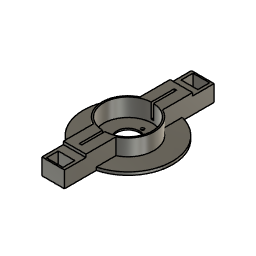
silnik v1 v2 (Autodesk Fusion 360 design; units mm, degrees)
Autodesk Fusion 360 part; units mm, degrees
cylinder "CylinderPrimitive1" add diameter 35 height 1 placed x (1, 0, 0) y (0, 1, 0) z (0, 0, 1) at (0, 0, 0)
cylinder "CylinderPrimitive2" cut diameter 15.2 height -1 placed x (1, 0, 0) y (0, 1, 0) z (0, 0, 1) at (0, 0, 1)
sketch "Sketch3" plane through (0, 0, 1) normal (0, 0, 1) x (-1, 0, 0)
  circle A0 centre (0, 0) radius 7.6
  circle A1 centre (0, 0) radius 17.5
  circle A2 centre (0, 0) radius 17.5
  circle A3 centre (0, 0) radius 16.5
  line L0 (-7.6, -50) -> (7.6, -50)
  line L1 (7.6, -50) -> (7.6, 50)
  line L2 (7.6, 50) -> (-7.6, 50)
  line L3 (-7.6, 50) -> (-7.6, -50)
  dimension "d5" = 33
  dimension "d6" = 15.2
  dimension "d7" = 100
  dimension "d8" = 50
  dimension "d9" = 7.6
  constraint coincident A0.centre A1.centre
  constraint horizontal L0
  constraint vertical L1
  constraint horizontal L2
  constraint vertical L3
  measures "d5" diameter of A3
  measures "d6" distance of L0.start L0.end
  measures "d7" distance of L0.start L2.end
  measures "d8" distance of A0.centre L0
  measures "d9" distance of A0.centre L3
extrude "Extrude1" add sketch "Sketch3" against normal blind 1 contours A1 A2 L1 L2 L3
extrude "Extrude2" add sketch "Sketch3" against normal blind 1 contours A1 A2 L0 L1 L3
extrude "Extrude3" add sketch "Sketch3" along normal blind 10 contours A1 A2 A3 L1 L3 | A1 A2 A3 L1 | A1 A2 A3 L1 L3 | A1 A2 A3 L3
sketch "Sketch4" plane through (0, 0, 1) normal (0, 0, 1) x (-1, 0, 0)
  arc A0 (-7.6, -15.7636) -> (7.6, -15.7636) centre (0, 0) ccw
  line L0 (-7.6, -15.7636) -> (-7.6, -50)
  line L1 (-7.6, -50) -> (7.6, -50)
  line L2 (7.6, -50) -> (7.6, -15.7636)
  line L3 (5.6, -49.5) -> (-5.6, -49.5)
  line L4 (-5.6, -49.5) -> (-5.6, -11)
  line L5 (-5.6, -11) -> (5.6, -11)
  line L6 (5.6, -11) -> (5.6, -49.5)
  line L7 (-7.6, 50) -> (-7.6, 15.7636)
  line L8 (7.6, 15.7636) -> (7.6, 50)
  line L9 (7.6, 50) -> (-7.6, 50)
  dimension "d16" = 2
  dimension "d17" = 2
  dimension "d18" = 0.5
  constraint horizontal L3
  constraint vertical L4
  constraint horizontal L5
  constraint vertical L6
  measures "d16" distance of L2 L6
  measures "d17" distance of L0 L4
  measures "d18" distance of L1 L3
extrude "Extrude4" add sketch "Sketch4" along normal blind 10 contours A0 L0 L1 L2 L3 L4 L6
sketch "Sketch5" plane through (0, 0, 1) normal (0, 0, 1) x (-1, 0, 0)
  arc A0 (7.6, 15.7636) -> (-7.6, 15.7636) centre (0, 0) ccw
  line L0 (7.6, 15.7636) -> (7.6, 50)
  line L1 (7.6, 50) -> (-7.6, 50)
  line L2 (-7.6, 50) -> (-7.6, 15.7636)
  line L3 (-5.6, 49.5) -> (5.6, 49.5)
  line L4 (5.6, 49.5) -> (5.6, 12.5)
  line L5 (5.6, 12.5) -> (-5.6, 12.5)
  line L6 (-5.6, 12.5) -> (-5.6, 49.5)
  dimension "d25" = 2
  dimension "d26" = 2
  dimension "d27" = 0.5
  constraint horizontal L3
  constraint vertical L4
  constraint horizontal L5
  constraint vertical L6
  measures "d25" distance of L2 L6
  measures "d26" distance of L0 L4
  measures "d27" distance of L1 L3
extrude "Extrude5" add sketch "Sketch5" along normal blind 10 contours A0 L0 L1 L2 L3 L4 L6
sketch "Sketch6" plane through (0, 0, 11) normal (0, 0, 1) x (-1, 0, 0)
  arc A0 (5.6, 16.5798) -> (-5.6, 16.5798) centre (0, 0) ccw
  line L0 (-5.6, 16.5798) -> (-5.6, 49.5)
  line L1 (-5.6, 49.5) -> (5.6, 49.5)
  line L2 (5.6, 49.5) -> (5.6, 16.5798)
  arc A1 (-5.6, -16.5798) -> (5.6, -16.5798) centre (0, 0) ccw
  line L3 (5.6, -16.5798) -> (5.6, -49.5)
  line L4 (5.6, -49.5) -> (-5.6, -49.5)
  line L5 (-5.6, -49.5) -> (-5.6, -16.5798)
  circle A2 centre (0, 0) radius 16.5
  line L6 (7.6, 15.7636) -> (7.6, 50)
  line L7 (7.6, 50) -> (-7.6, 50)
  line L8 (-7.6, 50) -> (-7.6, 15.7636)
  arc A3 (-7.6, 15.7636) -> (-7.6, -15.7636) centre (0, 0) ccw
  line L9 (-7.6, -15.7636) -> (-7.6, -50)
  line L10 (-7.6, -50) -> (7.6, -50)
  line L11 (7.6, -50) -> (7.6, -15.7636)
  arc A4 (7.6, -15.7636) -> (7.6, 15.7636) centre (0, 0) ccw
  line L12 (-5.6, 41.5) -> (5.6, 41.5)
  line L13 (5.6, 41.5) -> (5.6, 16.5798)
  line L14 (5.6, 16.5798) -> (-5.6, 16.5798)
  line L15 (-5.6, 16.5798) -> (-5.6, 41.5)
  line L16 (-5.6, -16.5798) -> (5.6, -16.5798)
  line L17 (5.6, -16.5798) -> (5.6, -41.5)
  line L18 (5.6, -41.5) -> (-5.6, -41.5)
  line L19 (-5.6, -41.5) -> (-5.6, -16.5798)
  dimension "d30" = 8
  dimension "d31" = 8
  constraint horizontal L12
  constraint vertical L13
  constraint horizontal L14
  constraint vertical L15
  constraint coincident A0.start L2.end
  constraint coincident L0 L12.start
  constraint horizontal L16
  constraint vertical L17
  constraint horizontal L18
  constraint vertical L19
  constraint coincident L3 L17.end
  constraint coincident A1.start L5.end
  measures "d30" distance of L1 L12
  measures "d31" distance of L4 L18
extrude "Extrude6" add sketch "Sketch6" against normal blind 10 contours A1 L3 L5 L17 L18 L19
extrude "Extrude7" add sketch "Sketch6" against normal blind 10 contours A0 L0 L2 L12 L13 L15
sketch "Sketch7" plane through (0, 0, 11) normal (0, 0, 1) x (-1, 0, 0)
  line L0 (5.6, 41.5) -> (-5.6, 41.5)
  line L1 (-5.6, 41.5) -> (-5.6, 49.5)
  line L2 (-5.6, 49.5) -> (5.6, 49.5)
  line L3 (5.6, 49.5) -> (5.6, 41.5)
  line L4 (5.6, -41.5) -> (5.6, -49.5)
  line L5 (5.6, -49.5) -> (-5.6, -49.5)
  line L6 (-5.6, -49.5) -> (-5.6, -41.5)
  line L7 (-5.6, -41.5) -> (5.6, -41.5)
  circle A0 centre (0, 0) radius 16.5
  line L8 (7.6, 15.7636) -> (7.6, 50)
  line L9 (7.6, 50) -> (-7.6, 50)
  line L10 (-7.6, 50) -> (-7.6, 15.7636)
  arc A1 (-7.6, 15.7636) -> (-7.6, -15.7636) centre (0, 0) ccw
  line L11 (-7.6, -15.7636) -> (-7.6, -50)
  line L12 (-7.6, -50) -> (7.6, -50)
  line L13 (7.6, -50) -> (7.6, -15.7636)
  arc A2 (7.6, -15.7636) -> (7.6, 15.7636) centre (0, 0) ccw
  line L14 (-2.5, -40.5) -> (-0.5, -40.5)
  line L15 (-0.5, -40.5) -> (-0.5, -17)
  line L16 (-0.5, -17) -> (-2.5, -17)
  line L17 (-2.5, -17) -> (-2.5, -40.5)
  line L18 (0.5, -40.5) -> (2.5, -40.5)
  line L19 (2.5, -40.5) -> (2.5, -17)
  line L20 (2.5, -17) -> (0.5, -17)
  line L21 (0.5, -17) -> (0.5, -40.5)
  line L22 (-2.5, 17) -> (-0.5, 17)
  line L23 (-0.5, 17) -> (-0.5, 40.5)
  line L24 (-0.5, 40.5) -> (-2.5, 40.5)
  line L25 (-2.5, 40.5) -> (-2.5, 17)
  line L26 (0.5, 17) -> (2.5, 17)
  line L27 (2.5, 17) -> (2.5, 40.5)
  line L28 (2.5, 40.5) -> (0.5, 40.5)
  line L29 (0.5, 40.5) -> (0.5, 17)
  dimension "d36" = 1
  dimension "d37" = 1
  dimension "d38" = 7.1
  dimension "d39" = 7.1
  dimension "d40" = 1
  dimension "d41" = 17
  dimension "d42" = 17
  dimension "d43" = 17
  dimension "d44" = 1
  dimension "d45" = 1
  constraint horizontal L14
  constraint vertical L15
  constraint horizontal L16
  constraint vertical L17
  constraint horizontal L18
  constraint vertical L19
  constraint horizontal L20
  constraint vertical L21
  constraint horizontal L22
  constraint vertical L23
  constraint horizontal L24
  constraint vertical L25
  constraint horizontal L26
  constraint vertical L27
  constraint horizontal L28
  constraint vertical L29
  measures "d36" distance of L15 L21
  measures "d37" distance of L23 L29
  measures "d38" distance of L11 L15.end
  measures "d39" distance of L10 L23.end
  measures "d40" distance of L0 L24
  measures "d41" distance of A0.centre L22
  measures "d42" distance of A0.centre L26
  measures "d43" distance of A0.centre L16
  measures "d44" distance of L7 L14
  measures "d45" distance of L7 L18
extrude "Extrude8" add sketch "Sketch7" along normal blind 10 contours L14 L15 L16 L17 | L18 L19 L20 L21 | L22 L23 L24 L25 | L26 L27 L28 L29
delete_face "Usuń powierzchnię1" 3 faces at (1.8333, -32.6667, 21) (2.5, -32.6667, 14.3333) (1.1667, -40.5, 14.3333)
delete_face "Usuń powierzchnię2" 2 faces at (-1.8333, -40.5, 17.6667) (-0.5, -32.6667, 14.3333)
delete_face "Usuń powierzchnię3" 3 faces at (2.5, 24.8333, 17.6667) (1.8333, 24.8333, 21) (1.1667, 17, 14.3333)
delete_face "Usuń powierzchnię4" 2 faces at (-0.5, 24.8333, 17.6667) (-1.8333, 17, 17.6667)
sketch "Szkic8" plane through (0, 0, 0) normal (0, 0, 1) x (1, 0, 0)
  circle A0 centre (0, 0) radius 30
  dimension "d48" = 60
  constraint coincident A0.centre origin
  measures "d48" diameter of A0
sketch "Szkic9" plane through (0, 0, 0) normal (0, 0, -1) x (1, 0, 0)
  circle A0 centre (0, 0) radius 7.6
  arc A1 (-7.6, 15.7636) -> (-7.6, -15.7636) centre (0, 0) ccw
  line L0 (-7.6, -15.7636) -> (-7.6, -50)
  line L1 (-7.6, -50) -> (7.6, -50)
  line L2 (7.6, -50) -> (7.6, -15.7636)
  arc A2 (7.6, -15.7636) -> (7.6, 15.7636) centre (0, 0) ccw
  line L3 (7.6, 15.7636) -> (7.6, 50)
  line L4 (7.6, 50) -> (-7.6, 50)
  line L5 (-7.6, 50) -> (-7.6, 15.7636)
  circle A3 centre (0, 0) radius 30
  dimension "d49" = 60
  constraint concentric A0 A3
  measures "d49" diameter of A3
extrude "Wyciągnięcie proste9" add sketch "Szkic9" against normal blind 2 contours A1 L0 L5 A3 | L2 A2 L3 A3
sketch "Szkic10" plane through (0, 0, 11) normal (0, 0, 1) x (-1, 0, 0)
  circle A0 centre (0, 0) radius 16.5
  line L0 (-7.6, -50) -> (7.6, -50)
  line L1 (7.6, -50) -> (7.6, -15.7636)
  arc A1 (7.6, -15.7636) -> (7.6, 15.7636) centre (0, 0) ccw
  line L2 (7.6, 15.7636) -> (7.6, 50)
  line L3 (7.6, 50) -> (-7.6, 50)
  line L4 (-7.6, 50) -> (-7.6, 15.7636)
  arc A2 (-7.6, 15.7636) -> (-7.6, -15.7636) centre (0, 0) ccw
  line L5 (-7.6, -15.7636) -> (-7.6, -50)
  line L6 (-5.6, 49.5) -> (5.6, 49.5)
  line L7 (5.6, 49.5) -> (5.6, 41.5)
  line L8 (5.6, 41.5) -> (-5.6, 41.5)
  line L9 (-5.6, 41.5) -> (-5.6, 49.5)
  line L10 (-5.6, -41.5) -> (5.6, -41.5)
  line L11 (5.6, -41.5) -> (5.6, -49.5)
  line L12 (5.6, -49.5) -> (-5.6, -49.5)
  line L13 (-5.6, -49.5) -> (-5.6, -41.5)
  line L14 (0.8, 32) -> (-0.8, 32)
  line L15 (-0.8, 32) -> (-0.8, -32)
  line L16 (-0.8, -32) -> (0.8, -32)
  line L17 (0.8, -32) -> (0.8, 32)
  dimension "d52" = 1.6
  dimension "d53" = 64
  dimension "d54" = 18
  dimension "d55" = 6.8
  constraint horizontal L14
  constraint vertical L15
  constraint horizontal L16
  constraint vertical L17
  measures "d52" distance of L14.start L14.end
  measures "d53" distance of L14.start L16.end
  measures "d54" distance of L3 L14
  measures "d55" distance of L4 L15
sketch "Szkic11" plane through (0, 0, 11) normal (0, 0, 1) x (-1, 0, 0)
  line L0 (-7.6, 50) -> (-7.6, 15.7636)
  line L1 (7.6, 15.7636) -> (7.6, 50)
  line L2 (-7.6, 36) -> (7.6, 36)
  line L3 (7.6, 50) -> (-7.6, 50)
  line L4 (-7.6, -15.7636) -> (-7.6, -50)
  line L5 (7.6, -50) -> (7.6, -15.7636)
  line L6 (-7.6, -36) -> (7.6, -36)
  line L7 (-7.6, -50) -> (7.6, -50)
  dimension "d56" = 14
  dimension "d57" = 14
  constraint coincident L0 L2.start
  constraint coincident L1 L2.end
  constraint perpendicular L1 L2
  constraint coincident L4 L6.start
  constraint coincident L5 L6.end
  constraint perpendicular L5 L6
  measures "d56" distance of L2 L3
  measures "d57" distance of L6 L7
extrude "Wyciągnięcie proste10" add 1 faces at (-0.411, -33.1513, 11) along direction (0, 0, 1) blind 4
extrude "Wyciągnięcie proste11" cut sketch "Szkic11" along normal blind 4
extrude "Wyciągnięcie proste12" cut sketch "Szkic10" along normal blind 4 and the other way blind 6 contours A0 L14 L15 L17 | A0 L15 L16 L17
extrude "Wyciągnięcie proste13" cut 1 faces at (-5.3333, -27.9212, 15) along direction (0, 0, -1) blind 2
extrude "Wyciągnięcie proste14" cut 2 faces at (-0.0889, -26.8326, 5) (-0.0889, 26.8326, 5) along direction (0, 0, -1) blind 2
extrude "Wyciągnięcie proste15" add 1 faces at (-2.5333, -50, 7.3333) along direction (0, -1, 0) blind 0.5
extrude "Wyciągnięcie proste16" add 1 faces at (2.5333, 50, 7.3333) along direction (0, 1, 0) blind 0.5
sketch "Szkic12" plane through (0, 0, 1) normal (0, 0, 1) x (-1, 0, 0)
  circle A0 centre (0, 0) radius 16.5
  circle A1 centre (0, 0) radius 7.6
  circle A2 centre (0, -9.9) radius 1.1
  line L0 (0, -9.9) -> (8.5737, 4.95)
  line L1 (8.5737, 4.95) -> (-8.5737, 4.95)
  line L2 (-8.5737, 4.95) -> (0, -9.9)
  circle A3 centre (-8.5737, 4.95) radius 1.1
  circle A4 centre (8.5737, 4.95) radius 1.1
  dimension "d74" = 2.2
  dimension "d75" = 9.9
  dimension "d76" = 2.2
  dimension "d77" = 2.2
  constraint coincident A2.centre L0.start
  constraint coincident A0.centre A1.centre
  constraint coincident L1.end L2.start
  constraint coincident L0.end L1.start
  measures "d74" diameter of A2
  measures "d75" distance of A0.centre A2.centre
  measures "d76" diameter of A3
  measures "d77" diameter of A4
hole "Otwór1" at (0, 9.9, 1) direction (0, 0, -1) diameter 2.2 depth 5 tip angle 118
extrude "Wyciągnięcie proste17" cut sketch "Szkic12" against normal blind 3 contours L0 L1 A4 | L0 L1 A4
extrude "Wyciągnięcie proste18" cut sketch "Szkic12" against normal blind 30 contours L1 L2 A3 | L1 L2 A3
equation "d54 = ( ( 16.5 + 19.5 ) / 2 ) * 1 mm"
equation "d75 = 12 mm - 2.1 mm"
